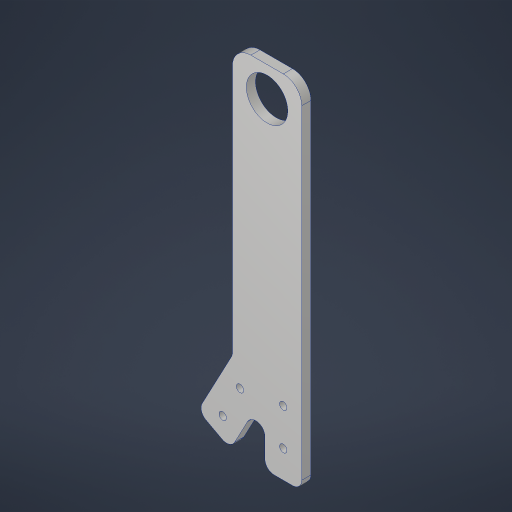
# Autodesk Inventor part: CL6-001
Saved by Autodesk Inventor 2023.4 (Build 274418000, 418)
## iProperties
Created: 2025-02-04
Part Number: CL6-001
Material: Aluminum 6061
Document SubType Name: Modeling
Designer: brand
Density: 2.7 g/cm^3
Appearance: Aluminum - Flat
Mass: 178.872 g
Surface Area: 256.07 cm^2
Volume: 66.2489 cm^3
Author: brand
Autodesk Inventor part; units mm, degrees
ref_plane "YZ Plane" through (0, 0, 0) normal (1, 0, 0) x (0, 1, 0)
ref_plane "XZ Plane" through (0, 0, 0) normal (0, 1, 0) x (-1, 0, 0)
ref_plane "XY Plane" through (0, 0, 0) normal (0, 0, 1) x (1, 0, 0)
sketch "Sketch1" plane through (0, 0, 0) normal (0, 0, 1) x (1, 0, 0)
  line L0 (-12.7, 0) -> (12.7, 0) construction
  line L1 (12.7, 0) -> (12.7, -57.15)
  line L2 (12.7, -57.15) -> (-12.7, -57.15)
  line L3 (-12.7, -57.15) -> (-12.7, 0) construction
  line L4 (-35.1269, 0) -> (-12.7, -11.9246) construction
  line L5 (-12.7, -11.9246) -> (-36.5492, -56.7783)
  line L6 (-36.5492, -56.7783) -> (-58.976, -44.8537)
  line L7 (-58.976, -44.8537) -> (-35.1269, 0)
  line L8 (-23.9134, -5.9623) -> (-47.7626, -50.816) construction
  line L9 (-35.1269, 0) -> (12.7, 0)
  line L10 (-12.7, -11.9246) -> (-12.7, -57.15)
  point P0 (0, 0)
  point P1 (0, 0)
  point P2 (-29.8757, -17.1757)
  point P3 (-41.8003, -39.6026)
  point P4 (0, -12.7)
  point P5 (0, -38.1)
  dimension "d0" = 25.4
  dimension "d1" = 25.4
  dimension "d2" = 28
  dimension "d3" = 50.8
  dimension "d4" = 25.4
  dimension "d5" = 12.7
  dimension "d6" = 25.4
  dimension "d7" = 12.7
  dimension "d8" = 57.15
  constraints: 22 end point, 4 perpendicular, 3 midpoint, 3 parallel, 3 point on line, 2 horizontal, 2 vertical alignment, 1 coincident, 1 horizontal alignment, 1 vertical
  measures "d0" distance of L1.end L2.end
  measures "d1" distance of L4.start L4.end
  measures "d2" angle of L3 L5
  measures "d3" distance of L8.start L8.end
  measures "d4" distance of point (-41.8, -39.603) point (-29.876, -17.176)
  measures "d5" distance from line of L4 point (-29.876, -17.176)
  measures "d6" distance of point (0, -38.1) point (0, -12.7)
  measures "d7" distance of point (0, 0) point (0, -12.7)
  measures "d8" distance of L0.end L1.end
extrude "Extrusion1" add sketch "Sketch1" against normal blind 6.35
hole "Hole1" at (-29.8757, -17.1757, 0) at (-41.8003, -39.6026, 0) at (0, -12.7, 0) at (0, -38.1, 0) direction (0, 0, -1) diameter 5.1054 end through all clearance for "Flat Head Machine Screw (82)" size "#10" standard "Ansi Unified Screw Threads"
sketch "Sketch2" plane through (0, 0, 0) normal (0, 0, 1) x (1, 0, 0)
  circle A0 centre (0, -12.7) radius 2.5527 construction
  circle A1 centre (-29.8757, -17.1757) radius 2.5527 construction
  circle A2 centre (-41.8003, -39.6026) radius 2.5527 construction
  circle A3 centre (0, -38.1) radius 2.5527 construction
  line L0 (-12.7, -57.15) -> (12.7, -57.15) construction
  line L1 (12.7, -57.15) -> (12.7, 0) construction
  line L2 (12.7, 0) -> (-35.1269, 0) projected
  line L3 (-35.1269, 0) -> (-58.976, -44.8537) construction
  line L4 (-58.976, -44.8537) -> (-36.5492, -56.7783) construction
  line L5 (-36.5492, -56.7783) -> (-12.7, -11.9246) construction
  line L6 (-12.7, -11.9246) -> (-12.7, -57.15) construction
  circle A4 centre (0, -12.7) radius 2.5527 construction
  circle A5 centre (-29.8757, -17.1757) radius 2.5527 construction
  circle A6 centre (-41.8003, -39.6026) radius 2.5527 construction
  circle A7 centre (0, -38.1) radius 2.5527 construction
  line L7 (12.7, 0) -> (12.7, -57.15) construction
  line L8 (12.7, -57.15) -> (-12.7, -57.15) construction
  line L9 (-12.7, -57.15) -> (-12.7, -11.9246) construction
  line L10 (-36.5492, -56.7783) -> (-58.976, -44.8537) construction
  line L11 (-58.976, -44.8537) -> (-35.1269, 0) construction
  line L12 (-35.1269, 0) -> (12.7, 0) construction
  circle A8 centre (-11.2134, 165.1) radius 14.2875 construction
  line L13 (12.7, 0) -> (-35.1269, 0) construction
  line L14 (-35.1269, 0) -> (-58.976, -44.8537) construction
  circle A9 centre (0, -12.7) radius 2.5527 construction
  circle A10 centre (-29.8757, -17.1757) radius 2.5527 construction
  circle A11 centre (-41.8003, -39.6026) radius 2.5527 construction
  circle A12 centre (0, -38.1) radius 2.5527 construction
  line L15 (12.7, 0) -> (12.7, -57.15) construction
  line L16 (12.7, -57.15) -> (-12.7, -57.15) construction
  line L17 (-12.7, -57.15) -> (-12.7, -11.9246) construction
  line L18 (-36.5492, -56.7783) -> (-58.976, -44.8537) construction
  line L19 (-58.976, -44.8537) -> (-35.1269, 0) construction
  line L20 (-35.1269, 0) -> (12.7, 0) construction
  line L21 (-35.1269, 0) -> (12.7, 0) construction
  line L22 (12.7, 0) -> (12.7, 185.7375)
  line L23 (12.7, 185.7375) -> (-35.1269, 185.7375)
  line L24 (-35.1269, 185.7375) -> (-35.1269, 0)
  line L25 (-12.7, -11.9246) -> (-36.5492, -56.7783) projected
  line L26 (-35.1269, 185.7375) -> (-31.8509, 185.7375)
  line L27 (-31.8509, 185.7375) -> (-31.8509, 144.4625)
  line L28 (-31.8509, 144.4625) -> (-35.1269, 144.4625)
  line L29 (-35.1269, 144.4625) -> (-35.1269, 185.7375)
  line L30 (-12.7, -11.9246) -> (-36.5492, -56.7783) projected
  point P0 (0, 0)
  point P1 (-11.2134, 0)
  point P2 (-11.2134, 0)
  point P3 (-11.2134, 179.3875)
  point P4 (-11.2134, 185.7375)
  point P5 (-11.2134, 150.8125)
  point P6 (-25.5009, 165.1)
  point P7 (-35.1269, 144.4625)
  dimension "d19" = 28.575
  dimension "d20" = 165.1
  dimension "d32" = 6.35
  dimension "d36" = 0
  dimension "d37" = 6.35
  dimension "d38" = 6.35
  constraints: 16 end point, 4 parallel, 3 midpoint, 3 point on circle, 2 horizontal, 2 perpendicular, 2 vertical alignment, 1 centre point, 1 coincident, 1 horizontal alignment
  measures "d19" diameter of A8
  measures "d20" distance from line of L2 A8.centre
  measures "d32" distance from line of L23 A8.start
  measures "d36" horizontal distance of point (-11.213, 185.738) A8.centre
  measures "d37" distance from line of point (-25.501, 165.1) L27
  measures "d38" distance from line of L28 A8.end
extrude "Extrusion2" add sketch "Sketch2" against normal up to surface (6.35 mm away)
fillet "Fillet1" radius 6.35 6 edges at (12.7, -57.15, -3.175) (-12.7, -57.15, -3.175) (-12.7, -11.9246, -3.175) (-36.5492, -56.7783, -3.175) (-58.976, -44.8537, -3.175) (-35.1269, 0, -3.175)
hole "Hole2" at (-11.2134, 165.1, 0) direction (0, 0, -1) diameter 28.575 end through all
fillet "Fillet2" radius 12.7 2 edges at (12.7, 185.7375, -3.175) (-35.1269, 185.7375, -3.175)
equation "\"d37\" = d32"
equation "\"d38\" = d32"
body "Solid1"
